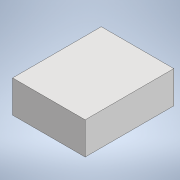
# Autodesk Inventor part: servo mg958 dummy
Saved by Autodesk Inventor 2020 (Build 240168000, 168)
## iProperties
Created: 2021-01-01
Part Number: servo mg958 dummy
Material: Generic
Document SubType Name: Modeling
Designer: Vikki
Density: 1 g/cm^3
Appearance: Copper - Polished
Author: Vikki
Autodesk Inventor part; units mm, degrees
ref_plane "YZ Plane" through (0, 0, 0) normal (1, 0, 0) x (0, 1, 0)
ref_plane "XZ Plane" through (0, 0, 0) normal (0, 1, 0) x (-1, 0, 0)
ref_plane "XY Plane" through (0, 0, 0) normal (0, 0, 1) x (1, 0, 0)
sketch "Sketch1" plane through (0, 0, 0) normal (0, 1, 0) x (-1, 0, 0)
  line L0 (0, 0) -> (45, 0)
  line L1 (45, 0) -> (45, -55)
  line L2 (45, -55) -> (0, -55)
  line L3 (0, -55) -> (0, 0)
  dimension "d0" = 45
  dimension "d1" = 55
  constraints: 8 end point, 2 parallel, 1 horizontal, 1 perpendicular
  measures "d0" distance between parallel lines of L3 L1
  measures "d1" distance of L0.end L1.end
extrude "Extrusion1" add sketch "Sketch1" along normal blind 20
sketch "Sketch2" plane through (-45, 0, -55) normal (-1, 0, 0) x (0, 0, 1)
  circle A0 centre (10, 10) radius 2.5
  line L0 (0, 0) -> (0, 20) projected
  line L1 (0, 0) -> (55, 0) projected
  dimension "d4" = 10
  dimension "d5" = 10
  dimension "d6" = 5
  constraints: 1 centre point
  measures "d4" distance from line of L0 A0.centre
  measures "d5" distance from line of L1 A0.centre
  measures "d6" diameter of A0
extrude "Extrusion2" add sketch "Sketch2" along normal blind 4
body "Solid1"
